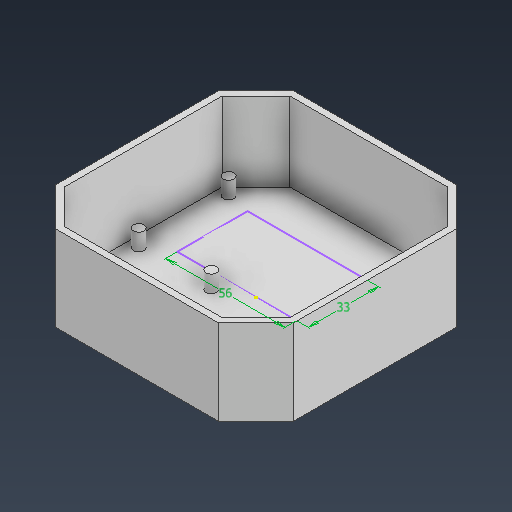
# Autodesk Inventor part: GPS-Compass_box
Saved by Autodesk Inventor 2026.2 (Build 302298000, 298)
## iProperties
Created: 2025-11-10
Part Number: GPS-Compass_box
Material: Generic
Document SubType Name: Modeling
Designer: MenMe
Density: 1 g/cm^3
Appearance: Default
Author: MenMe
Autodesk Inventor part; units mm, degrees
ref_plane "YZ Plane" through (0, 0, 0) normal (1, 0, 0) x (0, 1, 0)
ref_plane "XZ Plane" through (0, 0, 0) normal (0, 1, 0) x (-1, 0, 0)
ref_plane "XY Plane" through (0, 0, 0) normal (0, 0, 1) x (1, 0, 0)
sketch "Sketch1" plane through (0, 0, 0) normal (0, 1, 0) x (-1, 0, 0)
  line L0 (-56, 0) -> (56, 0) construction
  line L1 (0, 56) -> (0, -56) construction
  line L2 (56, 38.3223) -> (56, -38.3223)
  line L3 (56, 38.3223) -> (38.3223, 56)
  line L4 (38.3223, 56) -> (-38.3223, 56)
  line L5 (-38.3223, 56) -> (-56, 38.3223)
  line L6 (-56, 38.3223) -> (-56, -38.3223)
  line L7 (-56, -38.3223) -> (-38.3223, -56)
  line L8 (-38.3223, -56) -> (38.3223, -56)
  line L9 (38.3223, -56) -> (56, -38.3223)
  point P0 (0, 0)
  point P1 (0, 0)
  point P2 (56, 0)
  dimension "d0" = 112
  dimension "d1" = 112
  dimension "d2" = 135
  dimension "d3" = 135
  dimension "d4" = 135
  dimension "d8" = 25
  constraints: 20 end point, 7 midpoint, 2 horizontal, 2 perpendicular, 2 vertical, 1 coincident, 1 parallel
  measures "d0" distance of L0.start L0.end
  measures "d1" distance of L1.start L1.end
  measures "d2" angle of L2 L3
  measures "d3" angle of L2 L9
  measures "d4" angle of L5 L6
  measures "d8" distance of L6.end L7.end
extrude "Extrusion1" add sketch "Sketch1" along normal blind 40
sketch "Sketch2" plane through (0, 40, 0) normal (0, 1, 0) x (1, 0, 0)
  line L0 (38.3223, -56) -> (56, -38.3223) projected
  line L1 (56, -38.3223) -> (56, 38.3223) projected
  line L2 (56, 38.3223) -> (38.3223, 56) projected
  line L3 (38.3223, 56) -> (-38.3223, 56) projected
  line L4 (-38.3223, 56) -> (-56, 38.3223) projected
  line L5 (-56, 38.3223) -> (-56, -38.3223) projected
  line L6 (-56, -38.3223) -> (-38.3223, -56) projected
  line L7 (-38.3223, -56) -> (38.3223, -56) projected
  line L8 (-37.0797, 53) -> (37.0797, 53)
  line L9 (37.0797, 53) -> (53, 37.0797)
  line L10 (53, 37.0797) -> (53, -37.0797)
  line L11 (53, -37.0797) -> (37.0797, -53)
  line L12 (37.0797, -53) -> (-37.0797, -53)
  line L13 (-37.0797, -53) -> (-53, -37.0797)
  line L14 (-53, -37.0797) -> (-53, 37.0797)
  line L15 (-53, 37.0797) -> (-37.0797, 53)
  point P0 (0, 0)
  dimension "d11" = 3
  constraints: 16 end point, 7 other
  measures "d11" distance between parallel lines of L3 L8
extrude "Extrusion2" cut sketch "Sketch2" against normal blind 37 contours L8 L9 L10 L11 L12 L13 L14 L15
sketch "Sketch3" plane through (0, 3, 0) normal (0, 1, 0) x (1, 0, 0)
  circle A0 centre (-47.9582, 35.11) radius 2.5
  circle A1 centre (-47.9582, -7.09) radius 2.5
  circle A2 centre (-13.8582, -7.09) radius 2.5
  circle A3 centre (28.1418, 35.11) radius 2.5
  circle A4 centre (28.1418, 1.01) radius 2.5
  circle A5 centre (-14.0082, -33.0896) radius 2
  circle A6 centre (-47.8082, -33.0896) radius 2
  line L0 (-47.9582, -7.09) -> (-13.8582, -7.09) construction
  line L1 (-47.8082, -33.0896) -> (-14.0082, -33.0896) construction
  circle A7 centre (43.8518, 33.5) radius 2
  circle A8 centre (43.8518, -33.5) radius 2
  line L2 (37.0797, -53) -> (-37.0797, -53) projected
  line L3 (-53, -37.0797) -> (-53, 37.0797) projected
  line L4 (37.0797, 53) -> (53, 37.0797) projected
  line L5 (53, -37.0797) -> (37.0797, -53) projected
  line L6 (-10.6645, -2.1722) -> (28.1355, -2.1722)
  arc A9 (28.1355, -2.1722) -> (31.3355, 1.0278) centre (28.1355, 1.0278) ccw
  line L7 (31.3355, 35.1278) -> (31.3355, 1.0278)
  arc A10 (31.3355, 35.1278) -> (28.1355, 38.3278) centre (28.1355, 35.1278) ccw
  line L8 (6.8355, 38.3278) -> (28.1355, 38.3278)
  line L9 (6.8355, 32.6278) -> (6.8355, 38.3278)
  arc A11 (6.3355, 32.1278) -> (6.8355, 32.6278) centre (6.3355, 32.6278) ccw
  line L10 (-11.1645, 32.1278) -> (6.3355, 32.1278)
  arc A12 (-11.6645, 32.6278) -> (-11.1645, 32.1278) centre (-11.1645, 32.6278) ccw
  line L11 (-11.6645, 38.3278) -> (-11.6645, 32.6278)
  line L12 (-47.9645, 38.3278) -> (-11.6645, 38.3278)
  arc A13 (-47.9645, 38.3278) -> (-51.1645, 35.1278) centre (-47.9645, 35.1278) ccw
  line L13 (-51.1645, 35.1278) -> (-51.1645, 26.5778)
  arc A14 (-52.1645, 25.5778) -> (-51.1645, 26.5778) centre (-52.1645, 26.5778) ccw
  line L14 (-52.1645, 25.5778) -> (-52.6645, 25.5778)
  arc A15 (-52.6645, 25.5778) -> (-53.6645, 24.5778) centre (-52.6645, 24.5778) ccw
  line L15 (-53.6645, 24.5778) -> (-53.6645, 11.5778)
  arc A16 (-53.6645, 11.5778) -> (-52.6645, 10.5778) centre (-52.6645, 11.5778) ccw
  line L16 (-52.6645, 10.5778) -> (-52.1645, 10.5778)
  arc A17 (-51.1645, 9.5778) -> (-52.1645, 10.5778) centre (-52.1645, 9.5778) ccw
  line L17 (-51.1645, 9.5778) -> (-51.1645, -10.2722)
  line L18 (-51.1645, -10.2722) -> (-47.9645, -10.2722)
  arc A18 (-47.9645, -10.2722) -> (-44.7645, -7.0722) centre (-47.9645, -7.0722) ccw
  line L19 (-44.7645, -7.0722) -> (-44.7645, -6.6722)
  line L20 (-44.7645, -6.6722) -> (-17.0645, -6.6722)
  line L21 (-17.0645, -7.0722) -> (-17.0645, -6.6722)
  arc A19 (-17.0645, -7.0722) -> (-13.8645, -10.2722) centre (-13.8645, -7.0722) ccw
  line L22 (-13.8645, -10.2722) -> (-10.6645, -10.2722)
  line L23 (-10.6645, -2.1722) -> (-10.6645, -10.2722)
  line L24 (-51.1657, -10.3631) -> (-51.1657, -32.9831)
  arc A20 (-51.1657, -32.9831) -> (-47.8157, -36.3331) centre (-47.8157, -32.9831) ccw
  line L25 (-47.8157, -36.3331) -> (-14.0157, -36.3331)
  arc A21 (-14.0157, -36.3331) -> (-10.6657, -32.9831) centre (-14.0157, -32.9831) ccw
  line L26 (-10.6657, -10.3631) -> (-10.6657, -32.9831)
  line L27 (-10.6657, -10.3631) -> (-13.8657, -10.3631)
  arc A22 (-17.2157, -7.0131) -> (-13.8657, -10.3631) centre (-13.8657, -7.0131) ccw
  line L28 (-17.2157, -6.7631) -> (-17.2157, -7.0131)
  line L29 (-44.6157, -6.7631) -> (-17.2157, -6.7631)
  line L30 (-44.6157, -7.0131) -> (-44.6157, -6.7631)
  arc A23 (-47.9657, -10.3631) -> (-44.6157, -7.0131) centre (-47.9657, -7.0131) ccw
  line L31 (-51.1657, -10.3631) -> (-47.9657, -10.3631)
  arc A24 (38.8493, 37.5107) -> (36.8493, 35.5107) centre (38.8493, 35.5107) ccw
  line L32 (38.8493, 37.5107) -> (42.3493, 37.5107)
  line L33 (42.3493, 33.5107) -> (42.3493, 37.5107)
  arc A25 (42.3493, 33.5107) -> (45.3493, 33.5107) centre (43.8493, 33.5107) ccw
  line L34 (45.3493, 33.5107) -> (45.3493, 37.5107)
  line L35 (45.3493, 37.5107) -> (47.2531, 37.5107)
  line L36 (47.2531, 37.5107) -> (51.8493, 32.9145)
  line L37 (51.8493, -32.8931) -> (51.8493, 32.9145)
  line L38 (47.2531, -37.4893) -> (51.8493, -32.8931)
  line L39 (45.3493, -37.4893) -> (47.2531, -37.4893)
  line L40 (45.3493, -33.4893) -> (45.3493, -37.4893)
  arc A26 (45.3493, -33.4893) -> (42.3493, -33.4893) centre (43.8493, -33.4893) ccw
  line L41 (42.3493, -33.4893) -> (42.3493, -37.4893)
  line L42 (38.8493, -37.4893) -> (42.3493, -37.4893)
  arc A27 (36.8493, -35.4893) -> (38.8493, -37.4893) centre (38.8493, -35.4893) ccw
  line L43 (36.8493, 35.5107) -> (36.8493, -35.4893)
  point P0 (0, 0)
  point P1 (-30.9082, -33.0896)
  point P2 (-30.9082, -7.09)
  dimension "d40" = 5
  dimension "d43" = 34.1
  dimension "d58" = 76.1
  dimension "d59" = 42.2
  dimension "d60" = 34.1
  dimension "d90" = 33.8
  dimension "d105" = 26
  dimension "d128" = 4
  dimension "d135" = 67
  dimension "d144" = 34.51
  dimension "d147" = 15.71
  dimension "d264" = 9
  dimension "d265" = 9
  constraints: 80 end point, 38 point on circle, 28 centre point, 7 equal radius, 4 vertical alignment, 3 horizontal alignment, 2 horizontal, 2 midpoint
  measures "d40" diameter of A3
  measures "d43" distance of A3.centre A4.centre
  measures "d58" distance of A0.centre A3.centre
  measures "d59" distance of L0.start A0.centre
  measures "d60" distance of L0.end L0.start
  measures "d90" distance of L1.start L1.end
  measures "d105" distance of L1.end L0.end
  measures "d128" diameter of A5
  measures "d135" distance of A8.centre A7.centre
  measures "d144" vertical distance of A8.centre A4.centre
  measures "d147" horizontal distance of A7.centre A3.centre
  measures "d264" distance from line of L4 A7.centre
  measures "d265" distance from line of L5 A8.centre
extrude "Extrusion3" add sketch "Sketch3" along normal blind 8 contours A0 | A1 | A2 | A3 | A4 | A5 | A6 | A7 L33 A25 L34 | L34 A25 L33 A7 | L40 A26 L41 A8 | A8 L41 A26 L40
sketch "Sketch4" plane through (0, 3, 0) normal (0, 1, 0) x (1, 0, 0)
  line L0 (-37.1973, 33.2591) -> (18.8027, 33.2591)
  line L1 (18.8027, 33.2591) -> (18.8027, 0.2591)
  line L2 (18.8027, 0.2591) -> (-37.1973, 0.2591)
  line L3 (-37.1973, 0.2591) -> (-37.1973, 33.2591)
  point P0 (0, 0)
  dimension "d268" = 56
  dimension "d269" = 33
  constraints: 8 end point, 2 parallel, 1 horizontal, 1 perpendicular
  measures "d268" distance of L1.end L2.end
  measures "d269" distance of L0.end L1.end
body "Solid1"
